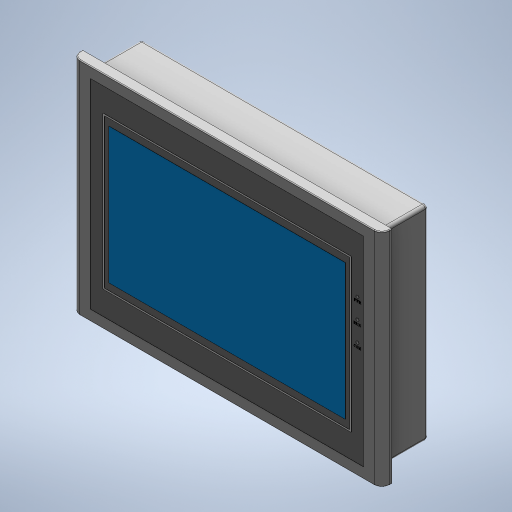
# Autodesk Inventor part: SANKOON  7 POL
Saved by Autodesk Inventor 2024 (Build 280153000, 153)
## iProperties
Created: 2022-09-08
Part Number: SANKOON  7 POL
Material: Genérico
Document SubType Name: Modeling
Designer: Tiago
Density: 1 g/cm^3
Appearance: Padrão
Item: 14
Quantidade: 01
Author: Tiago
Autodesk Inventor part; units mm, degrees
ref_plane "YZ Plane" through (0, 0, 0) normal (1, 0, 0) x (0, 1, 0)
ref_plane "XZ Plane" through (0, 0, 0) normal (0, 1, 0) x (-1, 0, 0)
ref_plane "XY Plane" through (0, 0, 0) normal (0, 0, 1) x (1, 0, 0)
sketch "Esboço8" plane through (0, 0, 0) normal (0, 0, 1) x (1, 0, 0)
  line L0 (-101.5, 72.5) -> (101.5, 72.5)
  line L1 (101.5, 72.5) -> (101.5, -72.5)
  line L2 (101.5, -72.5) -> (-101.5, -72.5)
  line L3 (-101.5, -72.5) -> (-101.5, 72.5)
  line L4 (-101.5, 72.5) -> (101.5, -72.5) construction
  line L5 (101.5, 72.5) -> (-101.5, -72.5) construction
  point P0 (0, 0)
  dimension "d24" = 203
  dimension "d25" = 145
  constraints: 12 end point, 2 midpoint, 2 parallel, 1 horizontal, 1 perpendicular
  measures "d24" distance of L0.start L0.end
  measures "d25" distance of L2.end L0.start
extrude "Extrusão6" add sketch "Esboço8" along normal blind 38
sketch "Esboço9" plane through (0, 0, 0) normal (0, 0, -1) x (-1, 0, 0)
  line L0 (-94, -67) -> (94, -67)
  line L1 (94, -67) -> (94, 67)
  line L2 (94, 67) -> (-94, 67)
  line L3 (-94, 67) -> (-94, -67)
  line L4 (-94, -67) -> (94, 67) construction
  line L5 (94, -67) -> (-94, 67) construction
  line L6 (-172.8736, 88.5977) -> (172.8736, 88.5977)
  line L7 (172.8736, 88.5977) -> (172.8736, -88.5977)
  line L8 (172.8736, -88.5977) -> (-172.8736, -88.5977)
  line L9 (-172.8736, -88.5977) -> (-172.8736, 88.5977)
  line L10 (-172.8736, 88.5977) -> (172.8736, -88.5977) construction
  line L11 (172.8736, 88.5977) -> (-172.8736, -88.5977) construction
  point P0 (0, 0)
  dimension "d28" = 188
  dimension "d29" = 134
  constraints: 24 end point, 4 midpoint, 4 parallel, 2 horizontal, 2 perpendicular
  measures "d28" distance of L1.end L2.end
  measures "d29" distance of L0.end L1.end
extrude "Extrusão7" cut sketch "Esboço9" against normal blind 31.5
sketch "Esboço11" plane through (0, 0, 0) normal (0, 0, -1) x (-1, 0, 0)
  line L0 (-94, -67) -> (94, -67) projected
  line L1 (-82, -67) -> (82, -67)
  line L2 (76, -42) -> (-76, -42)
  line L3 (-94, 67) -> (-94, -67) projected
  line L4 (94, -67) -> (94, 67) projected
  line L5 (76, -42) -> (82, -67)
  line L6 (-76, -42) -> (-82, -67)
  point P0 (0, 0)
  dimension "d40" = 25
  constraints: 8 end point, 1 horizontal, 1 parallel, 1 point on line
  measures "d40" distance between parallel lines of L0 L2
extrude "Extrusão9" cut sketch "Esboço11" against normal blind 23
fillet "Arredondamento1" radius 2 15 edges at (-94, 67, 15.75) (94, 67, 15.75) (94, -67, 15.75) (-94, -67, 15.75) (-94, 0, 0) (0, 67, 0) (94, 0, 0) (88, -67, 0) (79, -54.5, 0) (0, -42, 0) (82, -67, 11.5) (-82, -67, 11.5) (-79, -54.5, 0) (-88, -67, 0) (0, -67, 23)
sketch "Esboço13" plane through (0, 0, 38) normal (0, 0, 1) x (1, 0, 0)
  line L0 (-89.5, 65.5) -> (89.5, 65.5)
  line L1 (89.5, 65.5) -> (89.5, -65.5)
  line L2 (89.5, -65.5) -> (-89.5, -65.5)
  line L3 (-89.5, -65.5) -> (-89.5, 65.5)
  line L4 (-89.5, 65.5) -> (89.5, -65.5) construction
  line L5 (89.5, 65.5) -> (-89.5, -65.5) construction
  line L6 (-101.5, 72.5) -> (-101.5, -72.5) projected
  line L7 (101.5, 72.5) -> (-101.5, 72.5) projected
  point P0 (0, 0)
  dimension "d46" = 12
  dimension "d47" = 7
  constraints: 12 end point, 2 midpoint, 2 parallel, 1 horizontal, 1 perpendicular
  measures "d46" distance between parallel lines of L6 L3
  measures "d47" distance between parallel lines of L7 L0
extrude "Extrusão10" cut sketch "Esboço13" against normal blind 0.1
sketch "Esboço14" plane through (0, 0, 37.9) normal (0, 0, 1) x (1, 0, 0)
  line L0 (-77.5, 44.5) -> (77.5, 44.5)
  line L1 (77.5, 44.5) -> (77.5, -44.5)
  line L2 (77.5, -44.5) -> (-77.5, -44.5)
  line L3 (-77.5, -44.5) -> (-77.5, 44.5)
  line L4 (-77.5, 44.5) -> (77.5, -44.5) construction
  line L5 (77.5, 44.5) -> (-77.5, -44.5) construction
  line L6 (-89.5, -65.5) -> (-89.5, 65.5) projected
  line L7 (89.5, 65.5) -> (89.5, -65.5) projected
  line L8 (-89.5, 65.5) -> (89.5, 65.5) projected
  point P0 (0, 0)
  dimension "d50" = 12
  dimension "d51" = 12
  dimension "d52" = 21
  constraints: 12 end point, 2 midpoint, 2 parallel, 1 horizontal, 1 perpendicular
  measures "d50" distance between parallel lines of L6 L3
  measures "d51" distance between parallel lines of L7 L1
  measures "d52" distance between parallel lines of L8 L0
extrude "Extrusão11" add sketch "Esboço14" along normal blind 0.1
fillet "Arredondamento2" radius 5 2 edges at (-101.5, 0, 38) (101.5, 0, 38)
fillet "Arredondamento3" radius 0.5 10 edges at (-100.0355, 72.5, 36.5355) (-101.5, 72.5, 32.25) (100.0355, 72.5, 36.5355) (101.5, 72.5, 32.25) (0, 72.5, 38) (100.0355, -72.5, 36.5355) (101.5, -72.5, 32.25) (-100.0355, -72.5, 36.5355) (-101.5, -72.5, 32.25) (0, -72.5, 38)
sketch "Esboço15" plane through (0, 0, 37.9) normal (0, 0, 1) x (1, 0, 0)
  line L0 (80.5, -48.9725) -> (-80.5, -48.9725)
  line L1 (-80.5, -48.9725) -> (-80.5, 48.9725)
  line L2 (-80.5, 48.9725) -> (80.5, 48.9725)
  line L3 (80.5, 48.9725) -> (80.5, -48.9725)
  line L4 (80.5, -48.9725) -> (-80.5, 48.9725) construction
  line L5 (-80.5, -48.9725) -> (80.5, 48.9725) construction
  line L6 (-77.5, 44.5) -> (-77.5, -44.5) projected
  line L7 (-81.5, 49.9725) -> (-81.5, -49.9725)
  line L8 (-81.5, -49.9725) -> (81.5, -49.9725)
  line L9 (81.5, -49.9725) -> (81.5, 49.9725)
  line L10 (81.5, 49.9725) -> (-81.5, 49.9725)
  point P0 (0, 0)
  dimension "d57" = 3
  dimension "d58" = 1
  constraints: 20 end point, 4 parallel, 2 midpoint, 2 perpendicular, 1 horizontal, 3 other
  measures "d57" distance between parallel lines of L6 L1
  measures "d58" distance between parallel lines of L1 L7
extrude "Extrusão12" add sketch "Esboço15" along normal blind 0.1
fillet "Arredondamento4" radius 0.5 8 edges at (-81.5, 49.9725, 37.95) (-80.5, 48.9725, 37.95) (-81.5, -49.9725, 37.95) (-80.5, -48.9725, 37.95) (81.5, -49.9725, 37.95) (80.5, -48.9725, 37.95) (81.5, 49.9725, 37.95) (80.5, 48.9725, 37.95)
sketch "Esboço16" plane through (0, 0, 37.9) normal (0, 0, 1) x (1, 0, 0)
  circle A0 centre (85.5, 29) radius 1
  line L0 (83.1283, 27.3019) -> (92.6734, 27.3019) construction
  line L1 (92.6734, 27.3019) -> (92.6734, 24.2519) construction
  line L2 (92.6734, 24.2519) -> (83.1283, 24.2519) construction
  line L3 (83.1283, 24.2519) -> (83.1283, 27.3019) construction
  line L4 (89.5, 65.5) -> (89.5, -65.5) projected
  line L5 (82.8702, 14.2212) -> (92.4154, 14.2212) construction
  line L6 (92.4154, 14.2212) -> (92.4154, 11.1712) construction
  line L7 (92.4154, 11.1712) -> (82.8702, 11.1712) construction
  line L8 (82.8702, 11.1712) -> (82.8702, 14.2212) construction
  circle A1 centre (85.5, 16) radius 1
  circle A2 centre (85.5, 3) radius 1
  line L9 (82.9935, -1.7387) -> (82.9935, 1.3113) construction
  line L10 (82.9935, 1.3113) -> (92.5387, 1.3113) construction
  line L11 (92.5387, 1.3113) -> (92.5387, -1.7387) construction
  line L12 (92.5387, -1.7387) -> (82.9935, -1.7387) construction
  line L13 (84.4787, 26.7927) -> (84.406, 26.6459)
  line L14 (84.406, 26.6459) -> (84.3305, 26.5732)
  line L15 (84.3305, 26.5732) -> (84.1164, 26.5018)
  line L16 (84.1164, 26.5018) -> (83.6402, 26.5018)
  line L17 (83.6402, 26.5018) -> (83.6402, 25.9625)
  line L18 (83.6402, 25.9625) -> (83.6827, 25.876)
  line L19 (83.6827, 25.876) -> (83.7678, 25.8335)
  line L20 (83.7678, 25.8335) -> (83.8337, 25.8335)
  line L21 (83.8337, 25.8335) -> (83.8337, 25.8019)
  line L22 (83.8337, 25.8019) -> (83.2751, 25.8019)
  line L23 (83.2751, 25.8019) -> (83.2751, 25.8335)
  line L24 (83.2751, 25.8335) -> (83.341, 25.8335)
  line L25 (83.341, 25.8335) -> (83.4261, 25.876)
  line L26 (83.4261, 25.876) -> (83.4686, 25.9625)
  line L27 (83.4686, 25.9625) -> (83.4686, 27.1413)
  line L28 (83.4686, 27.1413) -> (83.4261, 27.2278)
  line L29 (83.4261, 27.2278) -> (83.341, 27.2703)
  line L30 (83.341, 27.2703) -> (83.2751, 27.2703)
  line L31 (83.2751, 27.2703) -> (83.2751, 27.3019)
  line L32 (83.2751, 27.3019) -> (84.1191, 27.3005)
  line L33 (84.1191, 27.3005) -> (84.3305, 27.2292)
  line L34 (84.3305, 27.2292) -> (84.406, 27.1564)
  line L35 (84.406, 27.1564) -> (84.4787, 27.0109)
  line L36 (84.4787, 27.0109) -> (84.4787, 26.7927)
  line L37 (84.3071, 26.7296) -> (84.3071, 27.0727)
  line L38 (84.3071, 27.0727) -> (84.2413, 27.2044)
  line L39 (84.2413, 27.2044) -> (84.1095, 27.2689)
  line L40 (84.1095, 27.2689) -> (83.7678, 27.2689)
  line L41 (83.7678, 27.2689) -> (83.6827, 27.2278)
  line L42 (83.6827, 27.2278) -> (83.6402, 27.1413)
  line L43 (83.6402, 27.1413) -> (83.6402, 26.5334)
  line L44 (83.6402, 26.5334) -> (84.1095, 26.5334)
  line L45 (84.1095, 26.5334) -> (84.2413, 26.5979)
  line L46 (84.2413, 26.5979) -> (84.3071, 26.7296)
  line L47 (86.293, 27.2703) -> (86.2257, 27.2703)
  line L48 (86.2257, 27.2703) -> (86.0967, 27.2058)
  line L49 (86.0967, 27.2058) -> (85.8168, 25.8019)
  line L50 (85.8168, 25.8019) -> (85.7907, 25.8019)
  line L51 (85.7907, 25.8019) -> (85.5244, 27.2003)
  line L52 (85.5244, 27.2003) -> (85.2582, 25.8019)
  line L53 (85.2582, 25.8019) -> (85.2307, 25.8019)
  line L54 (85.2307, 25.8019) -> (84.9673, 27.1921)
  line L55 (84.9673, 27.1921) -> (84.9206, 27.2388)
  line L56 (84.9206, 27.2388) -> (84.8232, 27.2703)
  line L57 (84.8232, 27.2703) -> (84.7545, 27.2703)
  line L58 (84.7545, 27.2703) -> (84.7545, 27.3019)
  line L59 (84.7545, 27.3019) -> (85.3145, 27.3019)
  line L60 (85.3145, 27.3019) -> (85.3145, 27.2703)
  line L61 (85.3145, 27.2703) -> (85.2486, 27.2703)
  line L62 (85.2486, 27.2703) -> (85.1621, 27.2278)
  line L63 (85.1621, 27.2278) -> (85.1402, 27.1825)
  line L64 (85.1402, 27.1825) -> (85.3117, 26.2616)
  line L65 (85.3117, 26.2616) -> (85.5038, 27.3019)
  line L66 (85.5038, 27.3019) -> (85.6781, 27.3019)
  line L67 (85.6781, 27.3019) -> (85.873, 26.252)
  line L68 (85.873, 26.252) -> (86.0651, 27.2086)
  line L69 (86.0651, 27.2086) -> (85.9403, 27.2703)
  line L70 (85.9403, 27.2703) -> (85.873, 27.2703)
  line L71 (85.873, 27.2703) -> (85.873, 27.3019)
  line L72 (85.873, 27.3019) -> (86.293, 27.3019)
  line L73 (86.293, 27.3019) -> (86.293, 27.2703)
  line L74 (87.7875, 25.9542) -> (87.7134, 25.8019)
  line L75 (87.7134, 25.8019) -> (87.5528, 25.8019)
  line L76 (87.5528, 25.8019) -> (87.4787, 25.9515)
  line L77 (87.4787, 25.9515) -> (87.3401, 26.3563)
  line L78 (87.3401, 26.3563) -> (87.2715, 26.5045)
  line L79 (87.2715, 26.5045) -> (87.1397, 26.5704)
  line L80 (87.1397, 26.5704) -> (86.8803, 26.5704)
  line L81 (86.8803, 26.5704) -> (86.8803, 25.9625)
  line L82 (86.8803, 25.9625) -> (86.9229, 25.876)
  line L83 (86.9229, 25.876) -> (87.008, 25.8335)
  line L84 (87.008, 25.8335) -> (87.0738, 25.8335)
  line L85 (87.0738, 25.8335) -> (87.0738, 25.8019)
  line L86 (87.0738, 25.8019) -> (86.5153, 25.8019)
  line L87 (86.5153, 25.8019) -> (86.5153, 25.8335)
  line L88 (86.5153, 25.8335) -> (86.5812, 25.8335)
  line L89 (86.5812, 25.8335) -> (86.6662, 25.876)
  line L90 (86.6662, 25.876) -> (86.7088, 25.9625)
  line L91 (86.7088, 25.9625) -> (86.7088, 27.1413)
  line L92 (86.7088, 27.1413) -> (86.6662, 27.2278)
  line L93 (86.6662, 27.2278) -> (86.5812, 27.2703)
  line L94 (86.5812, 27.2703) -> (86.5153, 27.2703)
  line L95 (86.5153, 27.2703) -> (86.5153, 27.3019)
  line L96 (86.5153, 27.3019) -> (87.3593, 27.3005)
  line L97 (87.3593, 27.3005) -> (87.5706, 27.2292)
  line L98 (87.5706, 27.2292) -> (87.6461, 27.1564)
  line L99 (87.6461, 27.1564) -> (87.7189, 27.0109)
  line L100 (87.7189, 27.0109) -> (87.7189, 26.8614)
  line L101 (87.7189, 26.8614) -> (87.6461, 26.7173)
  line L102 (87.6461, 26.7173) -> (87.5706, 26.6431)
  line L103 (87.5706, 26.6431) -> (87.3565, 26.5704)
  line L104 (87.3565, 26.5704) -> (87.2111, 26.5704)
  line L105 (87.2111, 26.5704) -> (87.2934, 26.532)
  line L106 (87.2934, 26.532) -> (87.3675, 26.4579)
  line L107 (87.3675, 26.4579) -> (87.5761, 26.0379)
  line L108 (87.5761, 26.0379) -> (87.6393, 25.9734)
  line L109 (87.6393, 25.9734) -> (87.6969, 25.9734)
  line L110 (87.6969, 25.9734) -> (87.7573, 26.0338)
  line L111 (87.7573, 26.0338) -> (87.7573, 26.0969)
  line L112 (87.7573, 26.0969) -> (87.7875, 26.0969)
  line L113 (87.7875, 26.0969) -> (87.7875, 25.9542)
  line L114 (87.5473, 26.801) -> (87.5473, 27.0727)
  line L115 (87.5473, 27.0727) -> (87.4814, 27.2044)
  line L116 (87.4814, 27.2044) -> (87.3497, 27.2689)
  line L117 (87.3497, 27.2689) -> (87.008, 27.2689)
  line L118 (87.008, 27.2689) -> (86.9229, 27.2278)
  line L119 (86.9229, 27.2278) -> (86.8803, 27.1413)
  line L120 (86.8803, 27.1413) -> (86.8803, 26.602)
  line L121 (86.8803, 26.602) -> (87.3497, 26.602)
  line L122 (87.3497, 26.602) -> (87.4814, 26.6692)
  line L123 (87.4814, 26.6692) -> (87.5473, 26.801)
  line L124 (84.2892, 12.8736) -> (84.2151, 12.7212)
  line L125 (84.2151, 12.7212) -> (84.0546, 12.7212)
  line L126 (84.0546, 12.7212) -> (83.9805, 12.8708)
  line L127 (83.9805, 12.8708) -> (83.8419, 13.2757)
  line L128 (83.8419, 13.2757) -> (83.7732, 13.4239)
  line L129 (83.7732, 13.4239) -> (83.6415, 13.4898)
  line L130 (83.6415, 13.4898) -> (83.3821, 13.4898)
  line L131 (83.3821, 13.4898) -> (83.3821, 12.8818)
  line L132 (83.3821, 12.8818) -> (83.4247, 12.7953)
  line L133 (83.4247, 12.7953) -> (83.5097, 12.7528)
  line L134 (83.5097, 12.7528) -> (83.5756, 12.7528)
  line L135 (83.5756, 12.7528) -> (83.5756, 12.7212)
  line L136 (83.5756, 12.7212) -> (83.0171, 12.7212)
  line L137 (83.0171, 12.7212) -> (83.0171, 12.7528)
  line L138 (83.0171, 12.7528) -> (83.0829, 12.7528)
  line L139 (83.0829, 12.7528) -> (83.168, 12.7953)
  line L140 (83.168, 12.7953) -> (83.2106, 12.8818)
  line L141 (83.2106, 12.8818) -> (83.2106, 14.0607)
  line L142 (83.2106, 14.0607) -> (83.168, 14.1471)
  line L143 (83.168, 14.1471) -> (83.0829, 14.1897)
  line L144 (83.0829, 14.1897) -> (83.0171, 14.1897)
  line L145 (83.0171, 14.1897) -> (83.0171, 14.2212)
  line L146 (83.0171, 14.2212) -> (83.8611, 14.2199)
  line L147 (83.8611, 14.2199) -> (84.0724, 14.1485)
  line L148 (84.0724, 14.1485) -> (84.1479, 14.0758)
  line L149 (84.1479, 14.0758) -> (84.2206, 13.9303)
  line L150 (84.2206, 13.9303) -> (84.2206, 13.7807)
  line L151 (84.2206, 13.7807) -> (84.1479, 13.6366)
  line L152 (84.1479, 13.6366) -> (84.0724, 13.5625)
  line L153 (84.0724, 13.5625) -> (83.8583, 13.4898)
  line L154 (83.8583, 13.4898) -> (83.7128, 13.4898)
  line L155 (83.7128, 13.4898) -> (83.7952, 13.4513)
  line L156 (83.7952, 13.4513) -> (83.8693, 13.3772)
  line L157 (83.8693, 13.3772) -> (84.0779, 12.9573)
  line L158 (84.0779, 12.9573) -> (84.141, 12.8928)
  line L159 (84.141, 12.8928) -> (84.1987, 12.8928)
  line L160 (84.1987, 12.8928) -> (84.2591, 12.9532)
  line L161 (84.2591, 12.9532) -> (84.2591, 13.0163)
  line L162 (84.2591, 13.0163) -> (84.2892, 13.0163)
  line L163 (84.2892, 13.0163) -> (84.2892, 12.8736)
  line L164 (84.0491, 13.7203) -> (84.0491, 13.992)
  line L165 (84.0491, 13.992) -> (83.9832, 14.1238)
  line L166 (83.9832, 14.1238) -> (83.8515, 14.1883)
  line L167 (83.8515, 14.1883) -> (83.5097, 14.1883)
  line L168 (83.5097, 14.1883) -> (83.4247, 14.1471)
  line L169 (83.4247, 14.1471) -> (83.3821, 14.0607)
  line L170 (83.3821, 14.0607) -> (83.3821, 13.5213)
  line L171 (83.3821, 13.5213) -> (83.8515, 13.5213)
  line L172 (83.8515, 13.5213) -> (83.9832, 13.5886)
  line L173 (83.9832, 13.5886) -> (84.0491, 13.7203)
  line L174 (85.9649, 14.1897) -> (85.899, 14.1897)
  line L175 (85.899, 14.1897) -> (85.7714, 14.1252)
  line L176 (85.7714, 14.1252) -> (85.7714, 13.1549)
  line L177 (85.7714, 13.1549) -> (85.6987, 12.9381)
  line L178 (85.6987, 12.9381) -> (85.5532, 12.794)
  line L179 (85.5532, 12.794) -> (85.3377, 12.7212)
  line L180 (85.3377, 12.7212) -> (85.1964, 12.7212)
  line L181 (85.1964, 12.7212) -> (85.1964, 12.735)
  line L182 (85.1964, 12.735) -> (85.1909, 12.7212)
  line L183 (85.1909, 12.7212) -> (84.9782, 12.794)
  line L184 (84.9782, 12.794) -> (84.8327, 12.9381)
  line L185 (84.8327, 12.9381) -> (84.7613, 13.1549)
  line L186 (84.7613, 13.1549) -> (84.7613, 14.0607)
  line L187 (84.7613, 14.0607) -> (84.7188, 14.1471)
  line L188 (84.7188, 14.1471) -> (84.6337, 14.1897)
  line L189 (84.6337, 14.1897) -> (84.5678, 14.1897)
  line L190 (84.5678, 14.1897) -> (84.5678, 14.2212)
  line L191 (84.5678, 14.2212) -> (85.1264, 14.2212)
  line L192 (85.1264, 14.2212) -> (85.1264, 14.1897)
  line L193 (85.1264, 14.1897) -> (85.0605, 14.1897)
  line L194 (85.0605, 14.1897) -> (84.9754, 14.1471)
  line L195 (84.9754, 14.1471) -> (84.9329, 14.0607)
  line L196 (84.9329, 14.0607) -> (84.9329, 13.089)
  line L197 (84.9329, 13.089) -> (85.0001, 12.8859)
  line L198 (85.0001, 12.8859) -> (85.066, 12.8214)
  line L199 (85.066, 12.8214) -> (85.2005, 12.7542)
  line L200 (85.2005, 12.7542) -> (85.3336, 12.7542)
  line L201 (85.3336, 12.7542) -> (85.5367, 12.8214)
  line L202 (85.5367, 12.8214) -> (85.6712, 12.9559)
  line L203 (85.6712, 12.9559) -> (85.7398, 13.159)
  line L204 (85.7398, 13.159) -> (85.7398, 14.1252)
  line L205 (85.7398, 14.1252) -> (85.6108, 14.1897)
  line L206 (85.6108, 14.1897) -> (85.545, 14.1897)
  line L207 (85.545, 14.1897) -> (85.545, 14.2212)
  line L208 (85.545, 14.2212) -> (85.9649, 14.2212)
  line L209 (85.9649, 14.2212) -> (85.9649, 14.1897)
  line L210 (87.6543, 14.1897) -> (87.5884, 14.1897)
  line L211 (87.5884, 14.1897) -> (87.4608, 14.1252)
  line L212 (87.4608, 14.1252) -> (87.4608, 12.7212)
  line L213 (87.4608, 12.7212) -> (87.4361, 12.7212)
  line L214 (87.4361, 12.7212) -> (86.4823, 14.1526)
  line L215 (86.4823, 14.1526) -> (86.4823, 12.8173)
  line L216 (86.4823, 12.8173) -> (86.6099, 12.7528)
  line L217 (86.6099, 12.7528) -> (86.6758, 12.7528)
  line L218 (86.6758, 12.7528) -> (86.6758, 12.7212)
  line L219 (86.6758, 12.7212) -> (86.2572, 12.7212)
  line L220 (86.2572, 12.7212) -> (86.2572, 12.7528)
  line L221 (86.2572, 12.7528) -> (86.3217, 12.7528)
  line L222 (86.3217, 12.7528) -> (86.4494, 12.8173)
  line L223 (86.4494, 12.8173) -> (86.4494, 14.1252)
  line L224 (86.4494, 14.1252) -> (86.3217, 14.1897)
  line L225 (86.3217, 14.1897) -> (86.2572, 14.1897)
  line L226 (86.2572, 14.1897) -> (86.2572, 14.2212)
  line L227 (86.2572, 14.2212) -> (86.614, 14.2212)
  line L228 (86.614, 14.2212) -> (87.4292, 12.9998)
  line L229 (87.4292, 12.9998) -> (87.4292, 14.1252)
  line L230 (87.4292, 14.1252) -> (87.3002, 14.1897)
  line L231 (87.3002, 14.1897) -> (87.2343, 14.1897)
  line L232 (87.2343, 14.1897) -> (87.2343, 14.2212)
  line L233 (87.2343, 14.2212) -> (87.6543, 14.2212)
  line L234 (87.6543, 14.2212) -> (87.6543, 14.1897)
  line L235 (84.274, 0.6965) -> (84.1751, 0.9957)
  line L236 (84.1751, 0.9957) -> (84.0379, 1.1302)
  line L237 (84.0379, 1.1302) -> (83.9048, 1.1974)
  line L238 (83.9048, 1.1974) -> (83.7031, 1.1974)
  line L239 (83.7031, 1.1974) -> (83.5686, 1.1315)
  line L240 (83.5686, 1.1315) -> (83.4341, 0.9284)
  line L241 (83.4341, 0.9284) -> (83.3655, 0.6526)
  line L242 (83.3655, 0.6526) -> (83.3655, 0.3068)
  line L243 (83.3655, 0.3068) -> (83.4341, 0.0309)
  line L244 (83.4341, 0.0309) -> (83.5686, -0.1722)
  line L245 (83.5686, -0.1722) -> (83.7031, -0.2381)
  line L246 (83.7031, -0.2381) -> (83.9048, -0.2381)
  line L247 (83.9048, -0.2381) -> (84.0379, -0.1708)
  line L248 (84.0379, -0.1708) -> (84.1751, -0.0336)
  line L249 (84.1751, -0.0336) -> (84.2438, 0.1036)
  line L250 (84.2438, 0.1036) -> (84.2726, 0.0885)
  line L251 (84.2726, 0.0885) -> (84.2026, -0.0542)
  line L252 (84.2026, -0.0542) -> (84.0585, -0.1969)
  line L253 (84.0585, -0.1969) -> (83.913, -0.2696)
  line L254 (83.913, -0.2696) -> (83.6934, -0.2683)
  line L255 (83.6934, -0.2683) -> (83.4821, -0.1969)
  line L256 (83.4821, -0.1969) -> (83.3353, -0.0542)
  line L257 (83.3353, -0.0542) -> (83.2666, 0.0899)
  line L258 (83.2666, 0.0899) -> (83.1939, 0.304)
  line L259 (83.1939, 0.304) -> (83.1939, 0.6567)
  line L260 (83.1939, 0.6567) -> (83.2666, 0.8708)
  line L261 (83.2666, 0.8708) -> (83.3353, 1.0149)
  line L262 (83.3353, 1.0149) -> (83.4821, 1.1576)
  line L263 (83.4821, 1.1576) -> (83.6948, 1.2304)
  line L264 (83.6948, 1.2304) -> (83.913, 1.2304)
  line L265 (83.913, 1.2304) -> (84.0585, 1.1576)
  line L266 (84.0585, 1.1576) -> (84.182, 1.0341)
  line L267 (84.182, 1.0341) -> (84.274, 1.3113)
  line L268 (84.274, 1.3113) -> (84.274, 0.6965)
  line L269 (85.8234, 0.3726) -> (85.7534, 0.0899)
  line L270 (85.7534, 0.0899) -> (85.6806, -0.0542)
  line L271 (85.6806, -0.0542) -> (85.5365, -0.1969)
  line L272 (85.5365, -0.1969) -> (85.3224, -0.2696)
  line L273 (85.3224, -0.2696) -> (85.1742, -0.2696)
  line L274 (85.1742, -0.2696) -> (85.1729, -0.2683)
  line L275 (85.1729, -0.2683) -> (84.9615, -0.1969)
  line L276 (84.9615, -0.1969) -> (84.8147, -0.0542)
  line L277 (84.8147, -0.0542) -> (84.7433, 0.0899)
  line L278 (84.7433, 0.0899) -> (84.6733, 0.3726)
  line L279 (84.6733, 0.3726) -> (84.6733, 0.5881)
  line L280 (84.6733, 0.5881) -> (84.7433, 0.8708)
  line L281 (84.7433, 0.8708) -> (84.8147, 1.0149)
  line L282 (84.8147, 1.0149) -> (84.9615, 1.1576)
  line L283 (84.9615, 1.1576) -> (85.1742, 1.2304)
  line L284 (85.1742, 1.2304) -> (85.3224, 1.2304)
  line L285 (85.3224, 1.2304) -> (85.3238, 1.229)
  line L286 (85.3238, 1.229) -> (85.5365, 1.1576)
  line L287 (85.5365, 1.1576) -> (85.6806, 1.0149)
  line L288 (85.6806, 1.0149) -> (85.7534, 0.8708)
  line L289 (85.7534, 0.8708) -> (85.8234, 0.5881)
  line L290 (85.8234, 0.5881) -> (85.8234, 0.3726)
  line L291 (85.6518, 0.3081) -> (85.6518, 0.6526)
  line L292 (85.6518, 0.6526) -> (85.5832, 0.9284)
  line L293 (85.5832, 0.9284) -> (85.4487, 1.1329)
  line L294 (85.4487, 1.1329) -> (85.3142, 1.1974)
  line L295 (85.3142, 1.1974) -> (85.1825, 1.1974)
  line L296 (85.1825, 1.1974) -> (85.048, 1.1329)
  line L297 (85.048, 1.1329) -> (84.9135, 0.9284)
  line L298 (84.9135, 0.9284) -> (84.8449, 0.6526)
  line L299 (84.8449, 0.6526) -> (84.8449, 0.3081)
  line L300 (84.8449, 0.3081) -> (84.9135, 0.0323)
  line L301 (84.9135, 0.0323) -> (85.048, -0.1722)
  line L302 (85.048, -0.1722) -> (85.1825, -0.2381)
  line L303 (85.1825, -0.2381) -> (85.3142, -0.2381)
  line L304 (85.3142, -0.2381) -> (85.4487, -0.1722)
  line L305 (85.4487, -0.1722) -> (85.5832, 0.0323)
  line L306 (85.5832, 0.0323) -> (85.6518, 0.3081)
  line L307 (87.7076, -0.2696) -> (87.1491, -0.2696)
  line L308 (87.1491, -0.2696) -> (87.1491, -0.2381)
  line L309 (87.1491, -0.2381) -> (87.2149, -0.2381)
  line L310 (87.2149, -0.2381) -> (87.3, -0.1955)
  line L311 (87.3, -0.1955) -> (87.3426, -0.1091)
  line L312 (87.3426, -0.1091) -> (87.3426, 1.1165)
  line L313 (87.3426, 1.1165) -> (86.8801, -0.2696)
  line L314 (86.8801, -0.2696) -> (86.8581, -0.2696)
  line L315 (86.8581, -0.2696) -> (86.3956, 1.1165)
  line L316 (86.3956, 1.1165) -> (86.3956, -0.1736)
  line L317 (86.3956, -0.1736) -> (86.5233, -0.2381)
  line L318 (86.5233, -0.2381) -> (86.5905, -0.2381)
  line L319 (86.5905, -0.2381) -> (86.5905, -0.2696)
  line L320 (86.5905, -0.2696) -> (86.1706, -0.2696)
  line L321 (86.1706, -0.2696) -> (86.1706, -0.2381)
  line L322 (86.1706, -0.2381) -> (86.2364, -0.2381)
  line L323 (86.2364, -0.2381) -> (86.3641, -0.1736)
  line L324 (86.3641, -0.1736) -> (86.3641, 1.1343)
  line L325 (86.3641, 1.1343) -> (86.2364, 1.1988)
  line L326 (86.2364, 1.1988) -> (86.1706, 1.1988)
  line L327 (86.1706, 1.1988) -> (86.1706, 1.2304)
  line L328 (86.1706, 1.2304) -> (86.5315, 1.2304)
  line L329 (86.5315, 1.2304) -> (86.9391, 0.0062)
  line L330 (86.9391, 0.0062) -> (87.3426, 1.2304)
  line L331 (87.3426, 1.2304) -> (87.7076, 1.2304)
  line L332 (87.7076, 1.2304) -> (87.7076, 1.1988)
  line L333 (87.7076, 1.1988) -> (87.6418, 1.1988)
  line L334 (87.6418, 1.1988) -> (87.5567, 1.1563)
  line L335 (87.5567, 1.1563) -> (87.5141, 1.0698)
  line L336 (87.5141, 1.0698) -> (87.5141, -0.1091)
  line L337 (87.5141, -0.1091) -> (87.5567, -0.1955)
  line L338 (87.5567, -0.1955) -> (87.6418, -0.2381)
  line L339 (87.6418, -0.2381) -> (87.7076, -0.2381)
  line L340 (87.7076, -0.2381) -> (87.7076, -0.2696)
  point P0 (0, 0)
  dimension "d62" = 2
  dimension "d63" = 4
  dimension "d65" = 2
  dimension "d66" = 13
  dimension "d67" = 2
  dimension "d68" = 13
  dimension "d69" = 3.05
  dimension "d70" = 3.05
  constraints: 3 centre point, 6 other
  measures "d62" diameter of A0
  measures "d63" distance from line of L4 A0.centre
  measures "d65" diameter of A1
  measures "d66" distance of A0.centre A1.centre
  measures "d67" diameter of A2
  measures "d68" distance of A1.centre A2.centre
  measures "d69" distance of L8.start L8.end
  measures "d70" distance of L9.start L9.end
extrude "Extrusão13" add sketch "Esboço16" along normal blind 0.1
